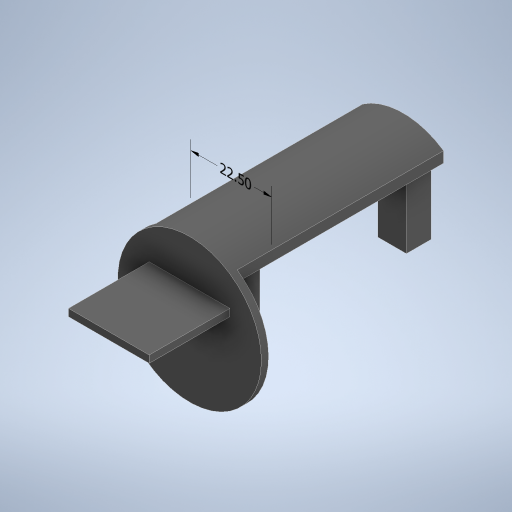
# Autodesk Inventor part: arm_2
Saved by Autodesk Inventor 2024.1 (Build 281209000, 209)
## iProperties
Created: 2025-01-27
Part Number: arm_2
Material: 一般
Document SubType Name: Modeling
Designer: hibik
Density: 1 g/cm^3
Appearance: 既定
Author: hibik
Autodesk Inventor part; units mm, degrees
ref_plane "YZ Plane" through (0, 0, 0) normal (1, 0, 0) x (0, 1, 0)
ref_plane "XZ Plane" through (0, 0, 0) normal (0, 1, 0) x (-1, 0, 0)
ref_plane "XY Plane" through (0, 0, 0) normal (0, 0, 1) x (1, 0, 0)
sketch "スケッチ1" plane through (0, 0, 0) normal (0, 1, 0) x (-1, 0, 0)
  line L0 (11.25, 0) -> (-11.25, 0)
  line L1 (-11.25, 0) -> (-11.25, -25)
  line L2 (-11.25, -25) -> (11.25, -25)
  line L3 (11.25, -25) -> (11.25, 0)
  point P0 (0, 0)
  point P1 (0, 0)
  dimension "d0" = 22.5
  dimension "d9" = 25
  constraints: 8 end point, 2 parallel, 1 coincident, 1 horizontal, 1 midpoint, 1 perpendicular
  measures "d0" distance of L0.start L0.end
  measures "d9" distance of L2.end L0.start
extrude "押し出し1" add sketch "スケッチ1" along normal blind 2
ref_plane "作業平面1" through (-11.25, 0, -22.5) normal (0, 0, 1) x (1, 0, 0)
sketch "スケッチ2" plane through (-11.25, 0, -22.5) normal (0, 0, 1) x (1, 0, 0)
  line L0 (0, 0) -> (0, 2) projected
  line L1 (0, 0) -> (22.5, 0)
  line L2 (22.5, 0) -> (22.5, -12.5)
  line L3 (22.5, -12.5) -> (0, -12.5)
  line L4 (0, -12.5) -> (0, 0)
  line L5 (22.5, 0) -> (22.5, 2) projected
  line L6 (0, -12.5) -> (22.5, -12.5)
  line L7 (22.5, -12.5) -> (22.5, -14.5)
  line L8 (22.5, -14.5) -> (0, -14.5)
  line L9 (0, -14.5) -> (0, -12.5)
  line L10 (0, 0) -> (22.5, -12.5) construction
  line L11 (22.5, 0) -> (0, -12.5) construction
  circle A0 centre (11.25, -6.25) radius 20
  point P0 (11.25, 0)
  dimension "d4" = 12.5
  dimension "d5" = 2
  dimension "d6" = 40
  constraints: 20 end point, 4 parallel, 2 collinear, 2 horizontal, 2 perpendicular, 1 centre point, 1 midpoint
  measures "d4" distance of L1.end L2.end
  measures "d5" distance of L6.end L7.end
  measures "d6" diameter of A0
extrude "押し出し2" add sketch "スケッチ2" against normal blind 2 contours L1 L2 L3 L4 | L3 L7 L8 L9 | A0
sketch "スケッチ3" plane through (0, 2, 0) normal (0, 1, 0) x (1, 0, 0)
  line L0 (-11.25, 24.5) -> (11.25, 24.5) projected
  line L1 (11.25, 24.5) -> (11.25, 25) projected
  line L2 (11.25, 25) -> (-11.25, 25) projected
  line L3 (-11.25, 25) -> (-11.25, 24.5) projected
  point P0 (0, 0)
extrude "押し出し3" add sketch "スケッチ3" along normal up to surface round surface about axis through (0, -6.25, -22.5) along (0, 0, -1) radius 20 far side no
sketch "スケッチ4" plane through (11.25, 0, -25) normal (0, 0, -1) x (-1, 0, 0)
  line L0 (0, 0) -> (22.5, 0) projected
  line L1 (22.5, 0) -> (22.5, 10.2859) projected
  arc A0 (22.5, 10.2859) -> (0, 10.2859) centre (11.25, -6.25) ccw projected
  line L2 (0, 0) -> (0, 10.2859) projected
  line L3 (0, 7.2859) -> (22.5, 7.2859)
  point P0 (11.25, 0)
  dimension "d12" = 3
  constraints: 2 end point, 2 point on line, 1 perpendicular
  measures "d12" distance from line of L1.end L3
extrude "押し出し4" add sketch "スケッチ4" along normal blind 57 contours L2 A0 L1 L3
ref_plane "作業平面2" through (7.8, 0, -24.5) normal (1, 0, 0) x (0, 0, -1)
sketch "スケッチ5" plane through (7.8, 0, -24.5) normal (1, 0, 0) x (0, 0, -1)
  line L0 (57.5, 7.2859) -> (57.5, 10.2859) projected
  line L1 (57.5, 7.2859) -> (2.9, 7.2859)
  line L2 (2.9, 7.2859) -> (2.9, -12.8141)
  line L3 (2.9, -12.8141) -> (57.5, -12.8141)
  line L4 (57.5, -12.8141) -> (57.5, 7.2859)
  line L5 (50.6, 7.2859) -> (9.8, 7.2859)
  line L6 (9.8, 7.2859) -> (9.8, -12.8141)
  line L7 (9.8, -12.8141) -> (50.6, -12.8141)
  line L8 (50.6, -12.8141) -> (50.6, 7.2859)
  line L9 (0.5, 0) -> (0.5, 7.2859) projected
  line L10 (0.5, 0) -> (2.9, 0)
  line L11 (0.5, 7.2859) -> (57.5, 7.2859) projected
  point P0 (-24.5, 0)
  point P1 (30.2, -12.8141)
  point P2 (30.2, -12.8141)
  point P3 (50.6, -12.8141)
  point P4 (9.8, -12.8141)
  point P5 (9.8, 7.2859)
  dimension "d19" = 54.6
  dimension "d20" = 40.8
  dimension "d21" = 20.1
  constraints: 18 end point, 4 parallel, 3 perpendicular, 2 horizontal, 2 midpoint, 2 point on line, 1 coincident, 1 collinear
  measures "d19" distance of L3.end L2.end
  measures "d20" distance of L7.end L6.end
  measures "d21" distance of L3.end L0.start
extrude "押し出し5" add sketch "スケッチ5" against normal blind 8 contours L4 L3 L8 L1 | L6 L3 L2 L1 | L2 L10 L9 L11
